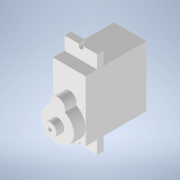
# Autodesk Inventor part: Microservo Mg90
Saved by Autodesk Inventor 2022 (Build 260153000, 153)
## iProperties
Created: 2021-09-13
Part Number: Microservo Mg90
Material: Generic
Document SubType Name: Modeling
Designer: Administrador
Density: 1 g/cm^3
Appearance: Default
Author: Administrador
Autodesk Inventor part; units mm, degrees
ref_plane "YZ Plane" through (0, 0, 0) normal (1, 0, 0) x (0, 1, 0)
ref_plane "XZ Plane" through (0, 0, 0) normal (0, 1, 0) x (-1, 0, 0)
ref_plane "XY Plane" through (0, 0, 0) normal (0, 0, 1) x (1, 0, 0)
sketch "Sketch1" plane through (0, 0, 0) normal (1, 0, 0) x (0, 1, 0)
  line L0 (7, 0) -> (29.5, 0)
  line L1 (0, 0) -> (7, 0)
  line L2 (7, 0) -> (29.5, 0)
  line L3 (29.5, 0) -> (29.5, 15.8)
  line L4 (7, 15.8) -> (7, 0)
  line L5 (29.5, 15.8) -> (34.4, 15.8) construction
  line L6 (2.1, 15.8) -> (2.1, 18.2)
  line L7 (34.4, 18.2) -> (34.4, 15.8)
  line L8 (7, 18.2) -> (7, 22.5)
  line L9 (7, 22.5) -> (29.5, 22.5)
  line L10 (29.5, 22.5) -> (29.5, 18.2)
  line L11 (2.1, 18.2) -> (7, 18.2)
  line L12 (29.5, 18.2) -> (34.4, 18.2)
  line L13 (34.4, 15.8) -> (29.5, 15.8)
  line L14 (7, 15.8) -> (2.1, 15.8)
  dimension "d2" = 22.5
  dimension "d3" = 15.8
  dimension "d5" = 2.4
  dimension "d6" = 4.3
  dimension "d7" = 22.5
  dimension "d8" = 4.3
  dimension "d9" = 2.4
  dimension "d10" = 15.8
  dimension "d13" = 4.9
  dimension "d14" = 4.9
  constraints: 30 end point, 7 perpendicular, 5 parallel, 3 horizontal, 1 vertical
  measures "d2" distance of L0.start L0.end
  measures "d3" distance of L0.end L3.end
  measures "d5" distance of L6.start L6.end
  measures "d6" distance of L8.start L8.end
  measures "d7" distance between parallel lines of L10 L8
  measures "d8" distance between parallel lines of L12 L9
  measures "d9" distance between parallel lines of L12 L5
  measures "d10" distance between parallel lines of L0 L14
  measures "d13" distance from line of L7.start L10
  measures "d14" distance from line of L8 L6.end
extrude "Extrusion1" add sketch "Sketch1" along normal blind 12
sketch "Sketch2" plane through (0, 7, 22.5) normal (0, 0, 1) x (1, 0, 0)
  line L0 (0, 22.5) -> (0, 0) projected
  line L1 (0, 0) -> (12, 0) projected
  line L2 (12, 22.5) -> (12, 0) projected
  line L3 (0, 22.5) -> (12, 22.5) projected
  line L4 (0, 0) -> (12, 0) projected
  line L5 (0, -4.9) -> (12, -4.9) projected
  circle A0 centre (6, 6) radius 0.7 construction
  circle A1 centre (6, 6) radius 2.4 construction
  line L6 (0, 0) -> (12, 0) projected
  arc A2 (3.371, 11.3933) -> (8.629, 11.3933) centre (6, 6) ccw
  line L7 (12, 0) -> (12, 22.5) projected
  arc A3 (8.629, 11.3933) -> (3.371, 11.3933) centre (6, 12.2) ccw
  point P0 (0, -7)
  dimension "d16" = 1.4
  dimension "d17" = 4.8
  dimension "d20" = 5.5
  dimension "d21" = 6
  dimension "d22" = 6.2
  constraints: 4 centre point, 4 point on circle, 2 coincident, 1 tangent
  measures "d16" diameter of A0
  measures "d17" diameter of A1
  measures "d20" diameter of A3
  measures "d21" distance from line of A0.centre L1
  measures "d22" distance of A3.centre A0.centre
extrude "Extrusion2" add sketch "Sketch2" along normal blind 4.3 contours A2 A3
sketch "Sketch3" plane through (0, 7, 26.8) normal (0, 0, 1) x (1, 0, 0)
  circle A0 centre (6, 6) radius 0.7
  circle A1 centre (6, 6) radius 2.4
  dimension "d25" = 1.4
  dimension "d26" = 4.8
  constraints: 2 centre point, 1 coincident
  measures "d25" diameter of A0
  measures "d26" diameter of A1
extrude "Extrusion3" add sketch "Sketch3" along normal blind 2.9
sketch "Sketch4" plane through (0, 29.5, 18.2) normal (0, 0, 1) x (1, 0, 0)
  line L0 (0, -22.5) -> (0, -27.4) projected
  line L1 (0, -27.4) -> (12, -27.4) projected
  line L2 (12, -22.5) -> (12, -27.4) projected
  line L3 (0, -22.5) -> (12, -22.5) projected
  line L4 (0, 4.9) -> (0, 0) projected
  line L5 (0, 0) -> (12, 0) projected
  line L6 (12, 4.9) -> (12, 0) projected
  line L7 (0, 4.9) -> (12, 4.9) projected
  line L8 (0, -16.5) -> (0, -22.5) projected
  line L9 (0, 0) -> (0, -16.5) projected
  line L10 (12, 0) -> (12, -16.5) projected
  line L11 (12, -16.5) -> (12, -22.5) projected
  line L12 (0, -22.5) -> (0, 0) projected
  line L13 (0, -11.25) -> (12, -11.25)
  arc A0 (5.3, 4.9) -> (6.7, 4.9) centre (6, 4.3343) ccw
  line L14 (5.3, 4.9) -> (6.7, 4.9)
  line L15 (0, 4.9) -> (12, 4.9) projected
  arc A1 (6.7, -27.4) -> (5.3, -27.4) centre (6, -26.8343) ccw
  line L16 (5.3, -27.4) -> (6.7, -27.4)
  point P0 (0, -29.5)
  point P1 (5.3, -27.4)
  dimension "d32" = 5.3
  dimension "d33" = 5.3
  dimension "d35" = 0.9
  constraints: 6 end point, 4 point on circle, 3 symmetric about line, 2 centre point, 1 collinear, 1 midpoint, 1 perpendicular, 1 point on line, 1 other
  measures "d32" distance of L6.start L14.end
  measures "d33" distance of L4.start L14.start
  measures "d35" radius of A0
extrude "Extrusion4" cut sketch "Sketch4" against normal up to surface (2.4 mm away) contours A1 L1 | L7 A0
body "Solid1"
